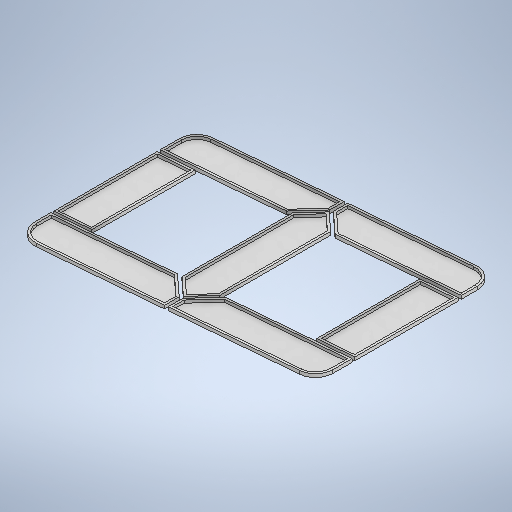
# Autodesk Inventor part: SegmentPanels
Saved by Autodesk Inventor 2025.2 (Build 292293000, 293)
## iProperties
Created: 2026-09-07
Part Number: SegmentPanels
Material: Generic
Document SubType Name: Modeling
Designer: Joefi
Density: 1 g/cm^3
Appearance: Default
Author: Joefi
Autodesk Inventor part; units mm, degrees
ref_plane "YZ Plane" through (0, 0, 0) normal (1, 0, 0) x (0, 1, 0)
ref_plane "XZ Plane" through (0, 0, 0) normal (0, 1, 0) x (-1, 0, 0)
ref_plane "XY Plane" through (0, 0, 0) normal (0, 0, 1) x (1, 0, 0)
sketch "Sketch1" plane through (0, 0, 0) normal (0, 1, 0) x (-1, 0, 0)
  line L0 (-20.8825, -45.9183) -> (-20.8825, 29.8831) construction
  line L1 (-20.8825, 29.8831) -> (-79.5857, 24.7472) construction
  line L2 (-79.5857, 24.7472) -> (-79.5857, -51.0541) construction
  line L3 (-79.5857, -51.0541) -> (-20.8825, -45.9183) construction
  circle A0 centre (-50.2341, -10.5855) radius 9 construction
  circle A1 centre (-50.2341, -10.5855) radius 9 construction
  line L4 (-20.8825, 29.8831) -> (-20.8825, -45.9183) construction
  line L5 (-20.8825, -45.9183) -> (-79.5857, -51.0541) construction
  line L6 (-79.5857, -51.0541) -> (-79.5857, 24.7472) construction
  line L7 (-79.5857, 24.7472) -> (-20.8825, 29.8831) construction
  circle A2 centre (38.4691, -2.825) radius 9 construction
  line L8 (9.1175, 32.5078) -> (67.8207, 37.6436) construction
  line L9 (67.8207, 37.6436) -> (67.8207, -38.1577) construction
  line L10 (67.8207, -38.1577) -> (9.1175, -43.2936) construction
  line L11 (9.1175, -43.2936) -> (9.1175, 32.5078) construction
  line L12 (-124.8825, 74.7073) -> (113.1175, 74.7073) construction
  arc A3 (117.1967, 70.6281) -> (113.1175, 74.7073) centre (113.1175, 70.6281) ccw construction
  line L13 (117.1967, 70.6281) -> (117.1967, -84.0386) construction
  arc A4 (113.1175, -88.1178) -> (117.1967, -84.0386) centre (113.1175, -84.0386) ccw construction
  line L14 (113.1175, -88.1178) -> (-124.8825, -88.1178) construction
  arc A5 (-128.9617, -84.0386) -> (-124.8825, -88.1178) centre (-124.8825, -84.0386) ccw construction
  line L15 (-128.9617, -84.0386) -> (-128.9617, 70.6281) construction
  arc A6 (-124.8825, 74.7073) -> (-128.9617, 70.6281) centre (-124.8825, 70.6281) ccw construction
  arc A7 (3.8039, -47.0078) -> (5.1175, -43.6299) centre (0.1175, -43.6299) ccw construction
  line L16 (5.1175, -43.6299) -> (5.1175, 31.8885) construction
  arc A8 (5.1175, 31.8885) -> (3.4954, 35.5748) centre (0.1175, 31.8885) ccw construction
  line L17 (3.4954, 35.5748) -> (-2.1961, 40.7902) construction
  arc A9 (-2.1961, 40.7902) -> (-9.2605, 40.4818) centre (-5.5741, 37.1038) ccw construction
  line L18 (-9.2605, 40.4818) -> (-15.5689, 33.5973) construction
  arc A10 (-15.5689, 33.5973) -> (-16.8825, 30.2194) centre (-11.8825, 30.2194) ccw construction
  line L19 (-16.8825, 30.2194) -> (-16.8825, -45.299) construction
  arc A11 (-16.8825, -45.299) -> (-15.2605, -48.9854) centre (-11.8825, -45.299) ccw construction
  line L20 (-15.2605, -48.9854) -> (-9.5689, -54.2007) construction
  arc A12 (-9.5689, -54.2007) -> (-2.5046, -53.8923) centre (-6.191, -50.5143) ccw construction
  line L21 (-2.5046, -53.8923) -> (3.8039, -47.0078) construction
  arc A13 (-2.8825, 51.7573) -> (-1.2605, 48.0709) centre (2.1175, 51.7573) ccw construction
  line L22 (-1.2605, 48.0709) -> (9.5259, 38.187) construction
  arc A14 (9.5259, 38.187) -> (13.3396, 36.8924) centre (12.9038, 41.8734) ccw construction
  line L23 (13.3396, 36.8924) -> (89.1727, 43.527) construction
  arc A15 (89.1727, 43.527) -> (93.7369, 48.5079) centre (88.7369, 48.5079) ccw construction
  line L24 (93.7369, 48.5079) -> (93.7369, 54.0059) construction
  arc A16 (93.7369, 54.0059) -> (81.7782, 64.9641) centre (82.7369, 54.0059) ccw construction
  line L25 (81.7782, 64.9641) -> (1.6817, 57.9565) construction
  arc A17 (1.6817, 57.9565) -> (-2.8825, 52.9756) centre (2.1175, 52.9756) ccw construction
  line L26 (-2.8825, 52.9756) -> (-2.8825, 51.7573) construction
  arc A18 (76.3849, 36.3853) -> (71.8207, 31.4043) centre (76.8207, 31.4043) ccw construction
  line L27 (71.8207, 31.4043) -> (71.8207, -30.3436) construction
  arc A19 (71.8207, -30.3436) -> (77.2564, -35.3246) centre (76.8207, -30.3436) ccw construction
  line L28 (77.2564, -35.3246) -> (89.1727, -34.282) construction
  arc A20 (89.1727, -34.282) -> (93.7369, -29.3011) centre (88.7369, -29.3011) ccw construction
  line L29 (93.7369, -29.3011) -> (93.7369, 32.4468) construction
  arc A21 (93.7369, 32.4468) -> (88.3012, 37.4278) centre (88.7369, 32.4468) ccw construction
  line L30 (88.3012, 37.4278) -> (76.3849, 36.3853) construction
  arc A22 (13.0849, -46.9618) -> (9.8343, -48.5648) centre (13.5207, -51.9428) ccw construction
  line L31 (9.8343, -48.5648) -> (-1.5689, -61.0092) construction
  arc A23 (-1.5689, -61.0092) -> (-2.8825, -64.3872) centre (2.1175, -64.3872) ccw construction
  line L32 (-2.8825, -64.3872) -> (-2.8825, -64.9862) construction
  arc A24 (-2.8825, -64.9862) -> (2.5533, -69.9672) centre (2.1175, -64.9862) ccw construction
  line L33 (2.5533, -69.9672) -> (83.6957, -62.8682) construction
  arc A25 (83.6957, -62.8682) -> (93.7369, -51.91) centre (82.7369, -51.91) ccw construction
  line L34 (93.7369, -51.91) -> (93.7369, -45.3622) construction
  arc A26 (93.7369, -45.3622) -> (88.3012, -40.3812) centre (88.7369, -45.3622) ccw construction
  line L35 (88.3012, -40.3812) -> (13.0849, -46.9618) construction
  arc A27 (-13.4467, -71.367) -> (-8.8825, -66.3861) centre (-13.8825, -66.3861) ccw construction
  line L36 (-8.8825, -66.3861) -> (-8.8825, -65.1678) construction
  arc A28 (-8.8825, -65.1678) -> (-10.5046, -61.4814) centre (-13.8825, -65.1678) ccw construction
  line L37 (-10.5046, -61.4814) -> (-21.2909, -51.5975) construction
  arc A29 (-21.2909, -51.5975) -> (-25.1046, -50.3029) centre (-24.6689, -55.2839) ccw construction
  line L38 (-25.1046, -50.3029) -> (-100.9378, -56.9375) construction
  arc A30 (-100.9378, -56.9375) -> (-105.502, -61.9184) centre (-100.502, -61.9184) ccw construction
  line L39 (-105.502, -61.9184) -> (-105.502, -67.4164) construction
  arc A31 (-105.502, -67.4164) -> (-93.5433, -78.3746) centre (-94.502, -67.4164) ccw construction
  line L40 (-93.5433, -78.3746) -> (-13.4467, -71.367) construction
  arc A32 (-88.1499, -49.7958) -> (-83.5857, -44.8148) centre (-88.5857, -44.8148) ccw construction
  line L41 (-83.5857, -44.8148) -> (-83.5857, 16.9331) construction
  arc A33 (-83.5857, 16.9331) -> (-89.0215, 21.9141) centre (-88.5857, 16.9331) ccw construction
  line L42 (-89.0215, 21.9141) -> (-100.9378, 20.8715) construction
  arc A34 (-100.9378, 20.8715) -> (-105.502, 15.8906) centre (-100.502, 15.8906) ccw construction
  line L43 (-105.502, 15.8906) -> (-105.502, -45.8573) construction
  arc A35 (-105.502, -45.8573) -> (-100.0662, -50.8383) centre (-100.502, -45.8573) ccw construction
  line L44 (-100.0662, -50.8383) -> (-88.1499, -49.7958) construction
  arc A36 (-24.85, 33.5513) -> (-21.5994, 35.1543) centre (-25.2857, 38.5322) ccw construction
  line L45 (-21.5994, 35.1543) -> (-10.1961, 47.5987) construction
  arc A37 (-10.1961, 47.5987) -> (-8.8825, 50.9767) centre (-13.8825, 50.9767) ccw construction
  line L46 (-8.8825, 50.9767) -> (-8.8825, 51.5757) construction
  arc A38 (-8.8825, 51.5757) -> (-14.3183, 56.5567) centre (-13.8825, 51.5757) ccw construction
  line L47 (-14.3183, 56.5567) -> (-95.4607, 49.4577) construction
  arc A39 (-95.4607, 49.4577) -> (-105.502, 38.4995) centre (-94.502, 38.4995) ccw construction
  line L48 (-105.502, 38.4995) -> (-105.502, 31.9517) construction
  arc A40 (-105.502, 31.9517) -> (-100.0662, 26.9707) centre (-100.502, 31.9517) ccw construction
  line L49 (-100.0662, 26.9707) -> (-24.85, 33.5513) construction
  line L50 (10.4456, 34.6316) -> (95.7369, 42.0936) construction
  line L51 (95.7369, 42.0936) -> (95.7369, 54.0059) construction
  arc A41 (95.7369, 54.0059) -> (81.6039, 66.9565) centre (82.7369, 54.0059) ccw construction
  line L52 (81.6039, 66.9565) -> (-4.8825, 59.3899) construction
  line L53 (-4.8825, 59.3899) -> (-4.8825, 48.6772) construction
  line L54 (-4.8825, 48.6772) -> (10.4456, 34.6316) construction
  line L55 (95.5619, 40.2463) -> (69.8054, 37.9929) construction
  line L56 (69.8054, 37.9929) -> (69.8054, -37.8084) construction
  line L57 (69.8054, -37.8084) -> (95.5619, -35.555) construction
  line L58 (95.5619, -35.555) -> (95.5619, 40.2463) construction
  line L59 (6.9425, -46.284) -> (6.9425, 34.8915) construction
  line L60 (6.9425, 34.8915) -> (-6.1241, 46.8649) construction
  line L61 (-6.1241, 46.8649) -> (-18.8825, 32.9415) construction
  line L62 (-18.8825, 32.9415) -> (-18.8825, -48.379) construction
  line L63 (-18.8825, -48.379) -> (-5.8882, -60.2862) construction
  line L64 (-5.8882, -60.2862) -> (6.9425, -46.284) construction
  line L65 (-22.0469, 31.9645) -> (-7.0575, 48.3226) construction
  line L66 (-7.0575, 48.3226) -> (-7.0575, 59.0392) construction
  line L67 (-7.0575, 59.0392) -> (-95.7948, 51.2757) construction
  arc A42 (-95.7948, 51.2757) -> (-107.502, 38.4995) centre (-94.677, 38.4995) ccw construction
  line L68 (-107.502, 38.4995) -> (-107.502, 24.4882) construction
  line L69 (-107.502, 24.4882) -> (-22.0469, 31.9645) construction
  line L70 (-7.0575, -62.1647) -> (-22.2721, -48.2231) construction
  line L71 (-22.2721, -48.2231) -> (-107.502, -55.6798) construction
  line L72 (-107.502, -55.6798) -> (-107.502, -67.4164) construction
  arc A43 (-107.502, -67.4164) -> (-93.5592, -80.1926) centre (-94.677, -67.4164) ccw construction
  line L73 (-93.5592, -80.1926) -> (-7.0575, -72.6247) construction
  line L74 (-7.0575, -72.6247) -> (-7.0575, -62.1647) construction
  line L75 (10.1988, -45.2066) -> (-4.8825, -61.665) construction
  line L76 (-4.8825, -61.665) -> (-4.8825, -72.4497) construction
  line L77 (-4.8825, -72.4497) -> (83.8547, -64.6862) construction
  arc A44 (83.8547, -64.6862) -> (95.5619, -51.91) centre (82.7369, -51.91) ccw construction
  line L78 (95.5619, -51.91) -> (95.5619, -37.7383) construction
  line L79 (95.5619, -37.7383) -> (10.1988, -45.2066) construction
  line L80 (-81.7607, -51.0688) -> (-81.7912, 24.7299) construction
  line L81 (-81.7912, 24.7299) -> (-107.5172, 22.4792) construction
  line L82 (-107.5172, 22.4792) -> (-107.5172, -53.3222) construction
  line L83 (-107.5172, -53.3222) -> (-81.7607, -51.0688) construction
  arc A45 (-95.8093, 53.4424) -> (-109.502, 38.4995) centre (-94.502, 38.4995) ccw construction
  line L84 (-95.8093, 53.4424) -> (81.4296, 68.9488) construction
  arc A46 (97.7369, 54.0059) -> (81.4296, 68.9488) centre (82.7369, 54.0059) ccw construction
  line L85 (97.7369, 54.0059) -> (97.7369, -51.91) construction
  arc A47 (84.0443, -66.853) -> (97.7369, -51.91) centre (82.7369, -51.91) ccw construction
  line L86 (84.0443, -66.853) -> (-93.1947, -82.3594) construction
  arc A48 (-109.502, -67.4164) -> (-93.1947, -82.3594) centre (-94.502, -67.4164) ccw construction
  line L87 (-109.502, -67.4164) -> (-109.502, 38.4995) construction
  arc A49 (107.1175, 70.6281) -> (113.1175, 64.6281) centre (113.1175, 70.6281) ccw construction
  line L88 (113.1175, 64.6281) -> (113.1175, -78.0386) construction
  arc A50 (113.1175, -78.0386) -> (107.1175, -84.0386) centre (113.1175, -84.0386) ccw construction
  line L89 (107.1175, -84.0386) -> (-118.8825, -84.0386) construction
  arc A51 (-118.8825, -84.0386) -> (-124.8825, -78.0386) centre (-124.8825, -84.0386) ccw construction
  line L90 (-124.8825, -78.0386) -> (-124.8825, 64.6281) construction
  arc A52 (-124.8825, 64.6281) -> (-118.8825, 70.6281) centre (-124.8825, 70.6281) ccw construction
  line L91 (-118.8825, 70.6281) -> (107.1175, 70.6281) construction
  line L92 (-4.8575, 59.367) -> (81.6061, 66.9316)
  arc A53 (95.7119, 54.0059) -> (81.6061, 66.9316) centre (82.7369, 54.0059) ccw
  line L93 (95.7119, 54.0059) -> (95.7119, 42.1165)
  line L94 (95.7119, 42.1165) -> (10.4543, 34.6575)
  line L95 (10.4543, 34.6575) -> (-4.8575, 48.6882)
  line L96 (-4.8575, 48.6882) -> (-4.8575, 59.367)
  line L97 (-4.8575, -61.6748) -> (10.2107, -45.2307)
  line L98 (10.2107, -45.2307) -> (95.5369, -37.7656)
  line L99 (95.5369, -37.7656) -> (95.5369, -51.91)
  arc A54 (83.8525, -64.6613) -> (95.5369, -51.91) centre (82.7369, -51.91) ccw
  line L100 (83.8525, -64.6613) -> (-4.8575, -72.4225)
  line L101 (-4.8575, -72.4225) -> (-4.8575, -61.6748)
  line L102 (-22.2808, -48.249) -> (-7.0825, -62.1757)
  line L103 (-7.0825, -62.1757) -> (-7.0825, -72.6018)
  line L104 (-7.0825, -72.6018) -> (-93.5614, -80.1677)
  arc A55 (-107.477, -67.4164) -> (-93.5614, -80.1677) centre (-94.677, -67.4164) ccw
  line L105 (-107.477, -67.4164) -> (-107.477, -55.7027)
  line L106 (-107.477, -55.7027) -> (-22.2808, -48.249)
  line L107 (6.9175, -46.2743) -> (6.9175, 34.8805)
  line L108 (6.9175, 34.8805) -> (-6.1226, 46.8295)
  line L109 (-6.1226, 46.8295) -> (-18.8575, 32.9318)
  line L110 (-18.8575, 32.9318) -> (-18.8575, -48.368)
  line L111 (-18.8575, -48.368) -> (-5.8897, -60.2508)
  line L112 (-5.8897, -60.2508) -> (6.9175, -46.2743)
  line L113 (-81.7857, -51.0458) -> (-81.8162, 24.7027)
  line L114 (-81.8162, 24.7027) -> (-107.4922, 22.4563)
  line L115 (-107.4922, 22.4563) -> (-107.4922, -53.2949)
  line L116 (-107.4922, -53.2949) -> (-81.7857, -51.0458)
  line L117 (-22.0588, 31.9886) -> (-7.0825, 48.3323)
  line L118 (-7.0825, 48.3323) -> (-7.0825, 59.0119)
  line L119 (-7.0825, 59.0119) -> (-95.7926, 51.2508)
  arc A56 (-95.7926, 51.2508) -> (-107.477, 38.4995) centre (-94.677, 38.4995) ccw
  line L120 (-107.477, 38.4995) -> (-107.477, 24.5155)
  line L121 (-107.477, 24.5155) -> (-22.0588, 31.9886)
  line L122 (95.5369, 40.2191) -> (69.8304, 37.97)
  line L123 (69.8304, 37.97) -> (69.8304, -37.7812)
  line L124 (69.8304, -37.7812) -> (95.5369, -35.5321)
  line L125 (95.5369, -35.5321) -> (95.5369, 40.2191)
  point P0 (0, 0)
  point P1 (-5.8825, -6.7053)
  dimension "d0" = 0.025
  dimension "d2" = 0.025
  dimension "d3" = 0.025
  dimension "d4" = 0.025
  dimension "d5" = 0.025
  dimension "d6" = 0.025
  dimension "d7" = 0.025
  constraints: 252 end point, 108 point on circle, 57 centre point, 31 other
  measures "d0" distance between parallel lines of L52 L92
  measures "d2" distance between parallel lines of L75 L97
  measures "d3" distance between parallel lines of L70 L102
  measures "d4" distance between parallel lines of L64 L112
  measures "d5" distance between parallel lines of L83 L116
  measures "d6" distance between parallel lines of L69 L121
  measures "d7" distance between parallel lines of L58 L125
extrude "Extrusion1" add sketch "Sketch1" along normal blind 0.4
sketch "Sketch2" plane through (0, 0.4, 0) normal (0, 1, 0) x (1, 0, 0)
  line L0 (-81.6061, -66.9316) -> (4.8575, -59.367) projected
  line L1 (4.8575, -59.367) -> (4.8575, -48.6882) projected
  line L2 (4.8575, -48.6882) -> (-10.4543, -34.6575) projected
  line L3 (-10.4543, -34.6575) -> (-95.7119, -42.1165) projected
  line L4 (-95.7119, -42.1165) -> (-95.7119, -54.0059) projected
  arc A0 (-95.7119, -54.0059) -> (-81.6061, -66.9316) centre (-82.7369, -54.0059) ccw projected
  line L5 (-94.1119, -43.5827) -> (-11.0162, -36.3127)
  line L6 (-11.0162, -36.3127) -> (3.2575, -49.3922)
  line L7 (3.2575, -49.3922) -> (3.2575, -57.9008)
  line L8 (3.2575, -57.9008) -> (-81.7455, -65.3376)
  arc A1 (-94.1119, -54.0059) -> (-81.7455, -65.3376) centre (-82.7369, -54.0059) ccw
  line L9 (-94.1119, -54.0059) -> (-94.1119, -43.5827)
  point P0 (0, 0)
  dimension "d10" = 1.6
  constraints: 10 end point, 2 point on circle, 1 centre point, 5 other
  measures "d10" distance between parallel lines of L3 L5
extrude "Extrusion2" add sketch "Sketch2" along normal blind 2
sketch "Sketch3" plane through (0, 0.4, 0) normal (0, 1, 0) x (1, 0, 0)
  line L0 (-69.8304, -37.97) -> (-69.8304, 37.7812) projected
  line L1 (-69.8304, 37.7812) -> (-95.5369, 35.5321) projected
  line L2 (-95.5369, 35.5321) -> (-95.5369, -40.2191) projected
  line L3 (-95.5369, -40.2191) -> (-69.8304, -37.97) projected
  line L4 (-71.4304, 36.0351) -> (-71.4304, -36.5039)
  line L5 (-71.4304, -36.5039) -> (-93.9369, -38.473)
  line L6 (-93.9369, -38.473) -> (-93.9369, 34.066)
  line L7 (-93.9369, 34.066) -> (-71.4304, 36.0351)
  point P0 (0, 0)
  dimension "d13" = 1.6
  constraints: 8 end point, 3 other
  measures "d13" distance between parallel lines of L0 L4
extrude "Extrusion3" add sketch "Sketch3" along normal blind 2
sketch "Sketch4" plane through (0, 0.4, 0) normal (0, 1, 0) x (1, 0, 0)
  line L0 (-95.5369, 51.91) -> (-95.5369, 37.7656) projected
  line L1 (-95.5369, 37.7656) -> (-10.2107, 45.2307) projected
  line L2 (-10.2107, 45.2307) -> (4.8575, 61.6748) projected
  line L3 (4.8575, 61.6748) -> (4.8575, 72.4225) projected
  line L4 (4.8575, 72.4225) -> (-83.8525, 64.6613) projected
  arc A0 (-83.8525, 64.6613) -> (-95.5369, 51.91) centre (-82.7369, 51.91) ccw projected
  line L5 (-10.97, 46.7704) -> (-93.9369, 39.5117)
  line L6 (-93.9369, 39.5117) -> (-93.9369, 51.91)
  arc A1 (-83.7131, 63.0674) -> (-93.9369, 51.91) centre (-82.7369, 51.91) ccw
  line L7 (-83.7131, 63.0674) -> (3.2575, 70.6764)
  line L8 (3.2575, 70.6764) -> (3.2575, 62.297)
  line L9 (3.2575, 62.297) -> (-10.97, 46.7704)
  point P0 (0, 0)
  dimension "d16" = 1.6
  constraints: 10 end point, 2 point on circle, 1 centre point, 5 other
  measures "d16" distance between parallel lines of L1 L5
extrude "Extrusion4" add sketch "Sketch4" along normal blind 2
sketch "Sketch5" plane through (0, 0.4, 0) normal (0, 1, 0) x (1, 0, 0)
  line L0 (-6.9175, -34.8805) -> (6.1226, -46.8295) projected
  line L1 (6.1226, -46.8295) -> (18.8575, -32.9318) projected
  line L2 (18.8575, -32.9318) -> (18.8575, 48.368) projected
  line L3 (18.8575, 48.368) -> (5.8897, 60.2508) projected
  line L4 (5.8897, 60.2508) -> (-6.9175, 46.2743) projected
  line L5 (-6.9175, 46.2743) -> (-6.9175, -34.8805) projected
  line L6 (17.2575, 47.664) -> (17.2575, -32.3096)
  line L7 (17.2575, -32.3096) -> (6.0239, -44.569)
  line L8 (6.0239, -44.569) -> (-5.3175, -34.1765)
  line L9 (-5.3175, -34.1765) -> (-5.3175, 45.652)
  line L10 (-5.3175, 45.652) -> (5.9884, 57.9903)
  line L11 (5.9884, 57.9903) -> (17.2575, 47.664)
  point P0 (0, 0)
  dimension "d19" = 1.6
  constraints: 12 end point, 5 other
  measures "d19" distance between parallel lines of L2 L6
extrude "Extrusion5" add sketch "Sketch5" along normal blind 2
sketch "Sketch6" plane through (0, 0.4, 0) normal (0, 1, 0) x (1, 0, 0)
  line L0 (7.0825, -48.3323) -> (7.0825, -59.0119) projected
  line L1 (7.0825, -59.0119) -> (95.7926, -51.2508) projected
  arc A0 (95.7926, -51.2508) -> (107.477, -38.4995) centre (94.677, -38.4995) ccw projected
  line L2 (107.477, -38.4995) -> (107.477, -24.5155) projected
  line L3 (107.477, -24.5155) -> (22.0588, -31.9886) projected
  line L4 (22.0588, -31.9886) -> (7.0825, -48.3323) projected
  line L5 (95.6531, -49.6569) -> (8.6825, -57.2659)
  line L6 (8.6825, -57.2659) -> (8.6825, -48.9545)
  line L7 (8.6825, -48.9545) -> (22.8181, -33.5283)
  line L8 (22.8181, -33.5283) -> (105.877, -26.2616)
  line L9 (105.877, -26.2616) -> (105.877, -38.4995)
  arc A1 (95.6531, -49.6569) -> (105.877, -38.4995) centre (94.677, -38.4995) ccw
  point P0 (0, 0)
  dimension "d22" = 1.6
  constraints: 10 end point, 2 point on circle, 1 centre point, 5 other
  measures "d22" distance between parallel lines of L1 L5
extrude "Extrusion6" add sketch "Sketch6" along normal blind 2
sketch "Sketch7" plane through (0, 0.4, 0) normal (0, 1, 0) x (1, 0, 0)
  line L0 (93.5614, 80.1677) -> (7.0825, 72.6018) projected
  line L1 (7.0825, 72.6018) -> (7.0825, 62.1757) projected
  line L2 (7.0825, 62.1757) -> (22.2808, 48.249) projected
  line L3 (22.2808, 48.249) -> (107.477, 55.7027) projected
  line L4 (107.477, 55.7027) -> (107.477, 67.4164) projected
  arc A0 (107.477, 67.4164) -> (93.5614, 80.1677) centre (94.677, 67.4164) ccw projected
  line L5 (105.877, 57.1688) -> (22.8427, 49.9043)
  line L6 (22.8427, 49.9043) -> (8.6825, 62.8797)
  line L7 (8.6825, 62.8797) -> (8.6825, 71.1357)
  line L8 (8.6825, 71.1357) -> (93.7008, 78.5738)
  arc A1 (105.877, 67.4164) -> (93.7008, 78.5738) centre (94.677, 67.4164) ccw
  line L9 (105.877, 67.4164) -> (105.877, 57.1688)
  point P0 (0, 0)
  dimension "d25" = 1.6
  constraints: 10 end point, 2 point on circle, 1 centre point, 5 other
  measures "d25" distance between parallel lines of L3 L5
extrude "Extrusion7" add sketch "Sketch7" along normal blind 2
sketch "Sketch8" plane through (0, 0.4, 0) normal (0, 1, 0) x (1, 0, 0)
  line L0 (81.8162, -24.7027) -> (107.4922, -22.4563) projected
  line L1 (107.4922, -22.4563) -> (107.4922, 53.2949) projected
  line L2 (107.4922, 53.2949) -> (81.7857, 51.0458) projected
  line L3 (81.7857, 51.0458) -> (81.8162, -24.7027) projected
  line L4 (105.8922, 51.5488) -> (105.8922, -20.9902)
  line L5 (105.8922, -20.9902) -> (83.4155, -22.9566)
  line L6 (83.4155, -22.9566) -> (83.3863, 49.5798)
  line L7 (83.3863, 49.5798) -> (105.8922, 51.5488)
  point P0 (0, 0)
  dimension "d28" = 1.6
  constraints: 8 end point, 3 other
  measures "d28" distance between parallel lines of L1 L4
extrude "Extrusion8" add sketch "Sketch8" along normal blind 2
equation "\"d0\" = d7"
equation "\"d2\" = d7"
equation "\"d3\" = d7"
equation "\"d4\" = d7"
equation "\"d5\" = d7"
equation "\"d6\" = d7"
body "Solid1"
